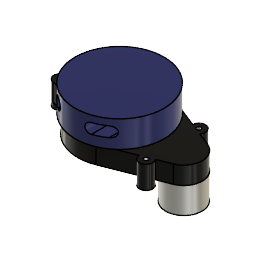
Lidar X2L (Autodesk Fusion 360 design; units mm, degrees)
Autodesk Fusion 360 part; units mm, degrees
note: some values were not read from the file. Set by a fixed rule: which sketch regions a step uses.
sketch "Sketch1" plane through (0, 0, 0) normal (0, 0, 1) x (1, 0, 0)
  circle A0 centre (0, 0) radius 30.25
  circle A1 centre (-40.3, 0) radius 4.5
  line L0 (-44.8, 0) -> (56.2, 0) construction
  circle A2 centre (36, 18) radius 4.5
  circle A3 centre (36, -18) radius 4.5
  line L1 (48.2764, -11.6322) -> (10.4348, -26.521)
  line L2 (48.2764, 11.6322) -> (10.4348, 26.521)
  circle A4 centre (43.7, 0) radius 12.4
  arc A5 (48.2764, -11.6322) -> (48.2764, 11.6322) centre (43.7, 0) ccw
  line L3 (-26, 0) -> (-26, 6.25) construction
  line L4 (-26, 6.25) -> (-27.8062, 6.25) construction
  line L5 (-28.4855, 6.1571) -> (-40.9096, 4.4585)
  line L6 (-28.4855, -6.1571) -> (-40.9096, -4.4585)
  arc A6 (10.4348, 26.521) -> (-27.6507, 6.9056) centre (0, 0) ccw
  arc A7 (-27.6507, -6.9056) -> (10.4348, -26.521) centre (0, 0) ccw
  arc A8 (-28.4855, 6.1571) -> (-27.6507, 6.9056) centre (-28.6209, 7.1479) ccw
  arc A9 (-27.6507, -6.9056) -> (-28.4855, -6.1571) centre (-28.6209, -7.1479) ccw
  line L7 (0, -32) -> (6, -32) construction
  line L8 (6, -32) -> (21, -32)
  line L9 (21, -32) -> (21, -12)
  line L10 (21, -12) -> (6, -12)
  line L11 (6, -12) -> (6, -32)
  line L12 (0, -32) -> (-13, -32) construction
  line L13 (-13, -32) -> (-21, -32)
  line L14 (-21, -32) -> (-21, -12)
  line L15 (-21, -12) -> (-13, -12)
  line L16 (-13, -12) -> (-13, -32)
  point P0 (-40.3, 0)
  dimension "d1" = 60.5
  dimension "d2" = 36
  dimension "d3" = 40.3
  dimension "d5" = 9
  dimension "d6" = 101
  dimension "d7" = 57
  dimension "d8" = 25
  dimension "d9" = 12.5
  dimension "d10" = 9
  dimension "d11" = 9
  dimension "d14" = 24.8
  dimension "d15" = 36
  dimension "d16" = 6.25
  dimension "d17" = 1
  dimension "d18" = 1
  dimension "d19" = 6
  dimension "d20" = 15
  dimension "d21" = 20
  dimension "d22" = 13
  dimension "d23" = 8
  dimension "d24" = 20
  constraint coincident A0.centre A6.centre
  constraint coincident P0 A1.centre
  constraint coincident A1 L0.start
  constraint horizontal L0
  constraint concentric A0 A6
  constraint coincident L0 A4.centre
  constraint tangent L1 A7
  constraint tangent L2 A6
  constraint concentric A4 A5
  constraint coincident L0 L3.start
  constraint perpendicular L0 L3
  constraint perpendicular L3 L4
  constraint coincident A1 L5.end
  constraint tangent A1 L5
  constraint symmetric L0 L5.end L6.end
  constraint concentric A6 A7
  constraint coincident L4.end L5
  constraint coincident L4.end A6
  constraint tangent L5 A8
  constraint tangent A6 A8
  constraint tangent L6 A9
  constraint tangent A7 A9
  constraint horizontal L7
  constraint horizontal L8
  constraint vertical L9
  constraint horizontal L10
  constraint vertical L11
  constraint parallel L7 L12
  constraint horizontal L13
  constraint vertical L14
  constraint horizontal L15
  constraint vertical L16
  measures "d1" diameter of A0
  measures "d2" distance of A2.centre A3.centre
  measures "d3" distance of A0.centre A1.centre
  measures "d5" diameter of A1
  measures "d6" distance of L0.start L0.end
  measures "d7" diameter of A6
  measures "d8" diameter of A5
  measures "d9" distance of L0.end A4.centre
  measures "d10" diameter of A2
  measures "d11" diameter of A3
  measures "d14" diameter of A4
  measures "d15" horizontal distance of A0.centre A2.centre
  measures "d16" distance of L3.start L3.end
  measures "d17" radius of A8
  measures "d18" radius of A9
  measures "d19" distance of L7.start L7.end
  measures "d20" distance of L7.end L8.end
  measures "d21" distance of L7.end L10.end
  measures "d22" distance of L7.start L12.end
  measures "d23" distance of L12.end L13.end
  measures "d24" distance of L12.end L15.end
extrude "Extrude1" add sketch "Sketch1" along normal blind 18 contours A0 L2 L5 L6 A6 A7 A8 A9 L9 L10 L11 L14 L15 L16 | A0 L2 L5 A6 A8 | A0 L1 A7 L9 L10 L11 | A0 L1 A7 L11 | A0 L6 A7 A9 L14 | A0 A7 L11 L16 | A0 A7 L14 L16 | A7 L14 L15 L16 makes body 1 in component "Scanner"
extrude "Extrude2" cut sketch "Sketch1" along normal mid plane 7 from surface at 10.1 contours A0 L1 A7 L9 L10 L11 | A0 L1 L8 L9 L11 | A0 L1 A7 L11 | A0 A7 L14 L16 | A0 L13 L14 L16 | A7 L14 L15 L16 bodies 1 in component "Scanner"
fillet "Fillet1" radius 3.5 8 edges at (21, -16.8865, 6.6) (21, -16.8865, 13.6) (6, -20.8245, 13.6) (6, -20.8245, 6.6) (-13, -19.6571, 6.6) (-13, -19.6571, 13.6) (-21, -16.8865, 13.6) (-21, -16.8865, 6.6) on bodies 1 in component "Scanner"
extrude "Extrude1'" add sketch "Sketch1" against normal blind 12 separate body contours A0 L2 L5 L6 A6 A7 A8 A9 L9 L10 L11 L14 L15 L16 | A0 A2 A3 L1 L2 A5 L9 | A0 L1 L9 | A0 L1 A7 L9 L10 L11 | A0 A1 L5 L6 | A7 L14 L15 L16 | A4 makes body 2 in component "Base"
extrude "Extrude2'" add sketch "Sketch1" against normal blind 15.5 contours A2 L2 | A2 L2 | A1 | A3 L1 | A3 L1 bodies 2 in component "Base"
extrude "Extrude3" add sketch "Sketch1" against normal blind 17.8 from surface at -12 contours A4 bodies 2 in component "Base"
hole "Hole1" at (-40.3, 0, 0) at (36, 18, 0) at (36, -18, 0) direction (0, 0, -1) diameter 2.93 end up to surface (15.5 mm away) bodies 2 in component "Base"
thread "Thread1" "ISO Metric profile 3.5 M3.5x0.6 M3.5x0.6 6H" thread offset 0 thread depth 7.4 in component "Base"
component "Base" placed x (1, 0, 0) y (0, 1, 0) z (0, 0, 1) at (0, 0, 0)
component "Scanner" placed x (1, 0, 0) y (0, 1, 0) z (0, 0, 1) at (0, 0, 0)
